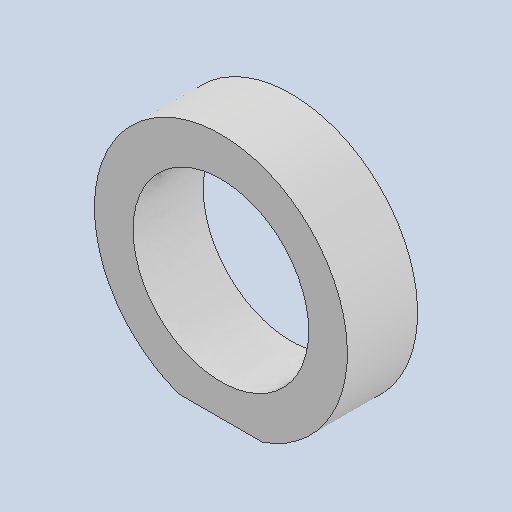
# Autodesk Inventor part: sleeve
Saved by Autodesk Inventor 2024.2 (Build 282272000, 272)
## iProperties
Created: 2024-06-01
Part Number: sleeve
Material: Generic
Document SubType Name: Modeling
Designer: user
Density: 1 g/cm^3
Appearance: Default
Author: user
Autodesk Inventor part; units mm, degrees
ref_plane "YZ Plane" through (0, 0, 0) normal (1, 0, 0) x (0, 1, 0)
ref_plane "XZ Plane" through (0, 0, 0) normal (0, 1, 0) x (-1, 0, 0)
ref_plane "XY Plane" through (0, 0, 0) normal (0, 0, 1) x (1, 0, 0)
sketch "Sketch2" plane through (0, 0, 0) normal (0, 0, 1) x (1, 0, 0)
  circle A0 centre (0, 0) radius 18
  circle A1 centre (0, 0) radius 12.5
  dimension "d0" = 36
  dimension "d1" = 25
  constraints: 2 centre point, 2 coincident
  measures "d0" diameter of A0
  measures "d1" diameter of A1
extrude "Extrusion1" add sketch "Sketch2" along normal mid plane 10
sketch "Sketch3" plane through (0, 0, 5) normal (0, 0, 1) x (1, 0, 0)
  circle A0 centre (0, 0) radius 18 projected
  line L0 (0, -25.2) -> (0, 25.2) projected
  line L1 (5.9161, -18) -> (-5.9161, -18)
  line L2 (-5.9161, -18) -> (-5.9161, -17)
  line L3 (-5.9161, -17) -> (5.9161, -17)
  line L4 (5.9161, -17) -> (5.9161, -18)
  point P0 (0, -18)
  point P1 (0, -17)
  dimension "d4" = 1
  constraints: 8 end point, 4 horizontal alignment, 2 parallel, 2 point on circle, 2 symmetric about line, 2 vertical alignment, 1 horizontal, 1 perpendicular
  measures "d4" distance of A0.start point (0, -17)
extrude "Extrusion2" cut sketch "Sketch3" against normal through all contours L4 L1 A0 | A0 L0 L3 | L1 L2 A0 | A0 L3 L0 picked at (3.3005, -17.1844) picked at (-3.3005, -17.1844)
body "Solid1"
